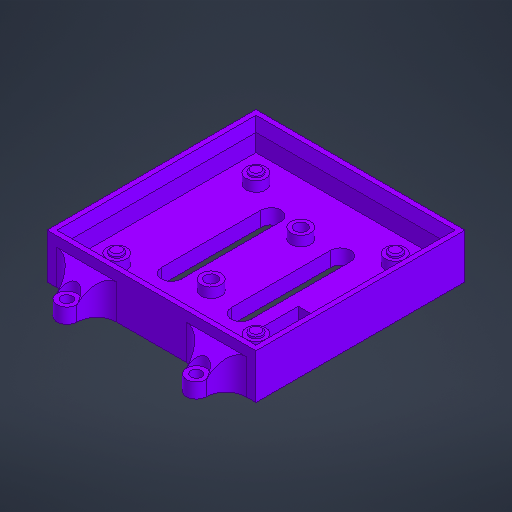
# Autodesk Inventor part: CameraMount
Saved by Autodesk Inventor 2025.1 (Build 291241000, 241)
## iProperties
Created: 2024-11-09
Part Number: CameraMount
Material: Generic
Document SubType Name: Modeling
Designer: jerem
Density: 1 g/cm^3
Appearance: Default
Author: jerem
## iProperties of the stored document CameraMount_3DPrint.ipt
Created: 2024-11-09
Part Number: CameraMount_3DPrint
Material: Generic
Document SubType Name: Modeling
Designer: jerem
Density: 1 g/cm^3
Appearance: Default
Author: jerem
Autodesk Inventor part; units mm, degrees
ref_plane "YZ Plane" through (0, 0, 0) normal (1, 0, 0) x (0, 1, 0)
ref_plane "XZ Plane" through (0, 0, 0) normal (0, 1, 0) x (-1, 0, 0)
ref_plane "XY Plane" through (0, 0, 0) normal (0, 0, 1) x (1, 0, 0)
sketch "Sketch1" plane through (0, 0, 0) normal (0, 1, 0) x (-1, 0, 0)
  line L0 (-21, -21) -> (21, -21)
  line L1 (21, -21) -> (21, 21)
  line L2 (21, 21) -> (-21, 21)
  line L3 (-21, 21) -> (-21, -21)
  line L4 (-21, -21) -> (21, 21) construction
  line L5 (21, -21) -> (-21, 21) construction
  line L6 (4.5, -4.5) -> (-4.5, 4.5) construction
  line L7 (-4.5, -4.5) -> (4.5, 4.5) construction
  circle A0 centre (14, 14) radius 1.3
  circle A1 centre (0, 9) radius 1.25
  circle A2 centre (-14, 14) radius 1.3
  circle A3 centre (0, -9) radius 1.25
  line L8 (0, 0) -> (0, 9) construction
  line L9 (0, -9) -> (0, 0) construction
  circle A4 centre (14, -14) radius 1.3
  circle A5 centre (-14, -14) radius 1.3
  line L10 (14, 14) -> (14, -14) construction
  line L11 (14, 14) -> (-14, 14) construction
  line L12 (-14, 14) -> (-14, -14) construction
  circle A6 centre (0, -9) radius 2
  circle A7 centre (0, 9) radius 2
  circle A8 centre (14, 14) radius 2
  circle A9 centre (-14, 14) radius 2
  circle A10 centre (-14, -14) radius 2
  circle A11 centre (14, -14) radius 2
  line L13 (-11.5, 3) -> (-15.5, 3)
  line L14 (-15.5, 3) -> (-15.5, 11)
  line L15 (-15.5, 11) -> (-11.5, 11)
  line L16 (-11.5, 11) -> (-11.5, 3)
  line L17 (19.5, 19.5) -> (19.5, -19.5)
  line L18 (19.5, -19.5) -> (-19.5, -19.5)
  line L19 (-19.5, -19.5) -> (-19.5, 19.5)
  line L20 (-19.5, 19.5) -> (19.5, 19.5)
  line L21 (-21, 3) -> (-21, -3)
  line L22 (21, -3) -> (21, 3)
  point P0 (0, 0)
  dimension "d0" = 42
  dimension "d1" = 42
  dimension "d2" = 9
  dimension "d3" = 2.5
  dimension "d4" = 2.5
  dimension "d5" = 9
  dimension "d6" = 9
  dimension "d7" = 2.6
  dimension "d8" = 2.6
  dimension "d9" = 2.6
  dimension "d10" = 2.6
  dimension "d11" = 28
  dimension "d14" = 4
  dimension "d15" = 4
  dimension "d16" = 4
  dimension "d17" = 4
  dimension "d18" = 4
  dimension "d19" = 4
  dimension "d20" = 8
  dimension "d21" = 4
  dimension "d26" = 11.5
  dimension "d27" = 3
  dimension "d28" = 1.5
  constraints: 47 end point, 12 centre point, 7 coincident, 6 parallel, 5 point on line, 4 midpoint, 4 vertical, 3 horizontal, 3 perpendicular, 3 other
  measures "d0" distance of L3.start L4.end
  measures "d1" distance of L0.end L4.end
  measures "d2" distance of L6.end L7.end
  measures "d3" diameter of A1
  measures "d4" diameter of A3
  measures "d5" distance of L9.end L9.start
  measures "d6" distance of L9.end L8.end
  measures "d7" diameter of A0
  measures "d8" diameter of A4
  measures "d9" diameter of A2
  measures "d10" diameter of A5
  measures "d11" distance of L11.start L12.start
  measures "d14" diameter of A6
  measures "d15" diameter of A7
  measures "d16" diameter of A8
  measures "d17" diameter of A9
  measures "d18" diameter of A10
  measures "d19" diameter of A11
  measures "d20" distance of L15.end L13.start
  measures "d21" distance of L13.start L13.end
  measures "d26" distance from line of point (0, 0) L16
  measures "d27" distance from line of point (0, 0) L13
  measures "d28" distance between parallel lines of L2 L20
extrude "Extrusion1" add sketch "Sketch1" against normal blind 3 contours L3 L2 L1 L0 | A0 | A2 | A4 | A5 | A6 | A7 | A8 | A9 | A10 | A11 | L17 L18 L19 L20
extrude "Extrusion2" add sketch "Sketch1" along normal blind 2 contours A0 | A2 | A4 | A5 | A6 | A7 | A8 | A9 | A10 | A11
extrude "Extrusion3" add sketch "Sketch1" along normal blind 6 contours L3 L2 L1 L0
sketch "Sketch2" plane through (0, -3, 0) normal (0, -1, 0) x (1, 0, 0)
  line L0 (2.4249, 9) -> (1.2124, 6.9)
  line L1 (1.2124, 6.9) -> (-1.2124, 6.9)
  line L2 (-1.2124, 6.9) -> (-2.4249, 9)
  line L3 (-2.4249, 9) -> (-1.2124, 11.1)
  line L4 (-1.2124, 11.1) -> (1.2124, 11.1)
  line L5 (1.2124, 11.1) -> (2.4249, 9)
  circle A0 centre (0, 9) radius 0.95
  line L6 (2.4249, -9) -> (1.2124, -11.1)
  line L7 (1.2124, -11.1) -> (-1.2124, -11.1)
  line L8 (-1.2124, -11.1) -> (-2.4249, -9)
  line L9 (-2.4249, -9) -> (-1.2124, -6.9)
  line L10 (-1.2124, -6.9) -> (1.2124, -6.9)
  line L11 (1.2124, -6.9) -> (2.4249, -9)
  circle A1 centre (0, -9) radius 0.95
  point P0 (0, 0)
  dimension "d31" = 4.2
  dimension "d32" = 1.9
  dimension "d33" = 4.2
  dimension "d34" = 1.9
  constraints: 24 end point, 6 coincident, 2 centre point, 2 horizontal, 26 other
  measures "d31" distance between parallel lines of L4 L1
  measures "d32" diameter of A0
  measures "d33" distance between parallel lines of L10 L7
  measures "d34" diameter of A1
extrude "Extrusion4" cut sketch "Sketch2" against normal blind 2.75
chamfer "Chamfer1" distance 0.9 angle 45 12 edges at (1.8187, -0.25, 10.05) (-1.8187, -0.25, 10.05) (0, -0.25, 6.9) (0, -0.25, 11.1) (1.8187, -0.25, 7.95) (-1.8187, -0.25, 7.95) (0, -0.25, -6.9) (-1.8187, -0.25, -7.95) (0, -0.25, -11.1) (1.8187, -0.25, -7.95) (1.8187, -0.25, -10.05) (-1.8187, -0.25, -10.05)
sketch "Sketch4" plane through (0, 0, 0) normal (0, 1, 0) x (-1, 0, 0)
  line L0 (-15, 21) -> (-11, 21)
  line L1 (-11, 21) -> (-11, 27)
  line L2 (-11, 27) -> (-15, 27)
  line L3 (-15, 27) -> (-15, 21)
  circle A0 centre (-13, 25) radius 1.1
  line L4 (-13, 25) -> (-13, 21) construction
  line L5 (0, -30.8) -> (0, 37.8) construction
  line L6 (29.4, 0) -> (-29.4, 0) construction
  line L7 (21, 21) -> (-21, 21) projected
  line L8 (-21, 21) -> (-21, -21) projected
  circle A1 centre (-13, 25) radius 2
  point P0 (-13, 27)
  dimension "d59" = 2.2
  dimension "d61" = 4
  dimension "d63" = 25
  dimension "d67" = 8
  dimension "d97" = 6
  constraints: 10 end point, 2 centre point, 2 midpoint, 2 parallel, 1 coincident, 1 horizontal, 1 perpendicular, 1 point on line, 1 tangent, 1 vertical
  measures "d59" diameter of A0
  measures "d61" distance of L1.end L2.end
  measures "d63" distance from line of L6 L4.start
  measures "d67" distance from line of L8 L4.start
  measures "d97" distance between parallel lines of L2 L7
extrude "Extrusion6" add sketch "Sketch4" against normal up to surface (3 mm away)
mirror "Mirror1" about plane through (0, 0, 0) normal (1, 0, 0) of "Extrusion6"
mirror "Mirror4" about plane through (0, 0, 0) normal (0, 0, 1) of "Extrusion6", "Mirror1"
chamfer "Chamfer4" distance 4 angle 45 4 edges at (13, 0, 21) (-13, 0, 21) (-13, 0, -21) (13, 0, -21)
extrude "Extrusion8" cut sketch "Sketch4" along normal through all contours A1
mirror "Mirror5" about plane through (0, 0, 0) normal (0, 0, 1) of "Extrusion8"
mirror "Mirror6" about plane through (0, 0, 0) normal (1, 0, 0) of "Extrusion8", "Mirror5"
chamfer "Chamfer5" distance 0.5 distance2 2.5 4 edges at (0, 6, -19.5) (19.5, 6, 0) (0, 6, 19.5) (-19.5, 6, 0) measured on face at (20, 6, 0) measured on face at (-20, 6, 0) measured on face at (0, 6, -20) measured on face at (0, 6, 20)
fillet "Fillet5" radius 4 8 edges at (11, 0.5, -21) (-11, 0.5, -21) (-15, 0.5, -21) (15, 0.5, -21) (-15, 0.5, 21) (-11, 0.5, 21) (11, 0.5, 21) (15, 0.5, 21)
extrude "Extrusion9" add sketch "Sketch1" along normal blind 0.6 from surface at 2 contours A0 | A2 | A4 | A5
chamfer "Chamfer6" distance 0.3 angle 45 4 edges at (15.3, 2.6, -14) (15.3, 2.6, 14) (-12.7, 2.6, 14) (-12.7, 2.6, -14)
sketch "Sketch5" plane through (0, 0, 0) normal (0, 1, 0) x (1, 0, 0)
  circle A0 centre (7, 10) radius 2
  circle A1 centre (7, -10) radius 2
  line L0 (7, 10) -> (7, -10) construction
  line L1 (5, 10) -> (5, -10)
  line L2 (9, -10) -> (9, 10)
  line L3 (0, 0) -> (7, 0) construction
  line L4 (0, 0) -> (0, 13.1293) construction
  circle A2 centre (-7, 10) radius 2
  line L5 (-9, -10) -> (-9, 10)
  circle A3 centre (-7, -10) radius 2
  line L6 (-5, 10) -> (-5, -10)
  line L7 (-7, 10) -> (-7, -10) construction
  point P0 (-7, 0)
  dimension "d91" = 20
  dimension "d92" = 4
  dimension "d93" = 7
  constraints: 16 end point, 8 point on circle, 7 symmetric about line, 4 centre point, 4 tangent, 1 equal radius, 1 horizontal, 1 midpoint, 1 vertical, 2 other
  measures "d91" distance of L0.start L0.end
  measures "d92" distance between parallel lines of L2 L1
  measures "d93" distance of L3.start L3.end
extrude "Extrusion10" cut sketch "Sketch5" against normal through all
fillet "Fillet6" radius 2 8 edges at (-15, -1.5, -27) (-11, -1.5, -27) (-15, -1.5, 27) (-11, -1.5, 27) (11, -1.5, 27) (15, -1.5, 27) (11, -1.5, -27) (15, -1.5, -27)
equation "\"d1\" = d0"
equation "\"d4\" = d3"
equation "\"d5\" = d6"
equation "\"d8\" = d7"
equation "\"d9\" = d7"
equation "\"d10\" = d7"
equation "\"d14\" = d15"
equation "\"d17\" = d16"
equation "\"d18\" = d16"
equation "\"d19\" = d16"
equation "\"d31\" = d33"
body "Solid1"
